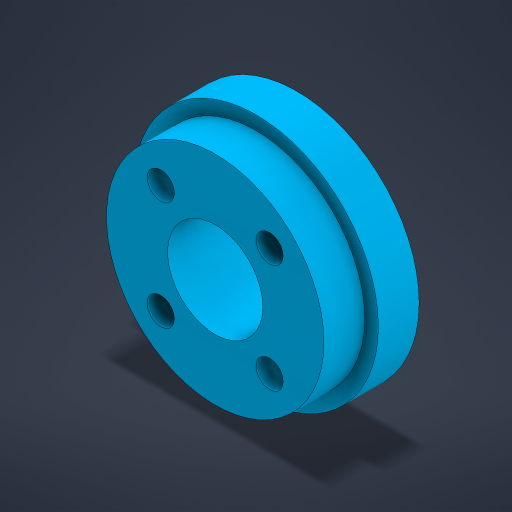
# Autodesk Inventor part: SecondStageArmClamp
Saved by Autodesk Inventor 2024 (Build 280153000, 153)
## iProperties
Created: 2024-01-28
Part Number: SecondStageArmClamp
Material: Generic
Document SubType Name: Modeling
Designer: avsar
Density: 1 g/cm^3
Appearance: Sky Blue Medium
Author: avsar
Autodesk Inventor part; units mm, degrees
ref_plane "YZ Plane" through (0, 0, 0) normal (1, 0, 0) x (0, 1, 0)
ref_plane "XZ Plane" through (0, 0, 0) normal (0, 1, 0) x (-1, 0, 0)
ref_plane "XY Plane" through (0, 0, 0) normal (0, 0, 1) x (1, 0, 0)
sketch "Sketch1" plane through (0, 0, 0) normal (0, 0, 1) x (1, 0, 0)
  circle A0 centre (0, 0) radius 18
  dimension "d0" = 36
  constraints: 1 centre point, 1 coincident
  measures "d0" diameter of A0
extrude "Extrusion1" add sketch "Sketch1" along normal blind 6
sketch "Sketch2" plane through (0, 0, 6) normal (0, 0, 1) x (1, 0, 0)
  circle A0 centre (0, 0) radius 16
  dimension "d3" = 32
  constraints: 1 centre point, 1 coincident
  measures "d3" diameter of A0
extrude "Extrusion2" add sketch "Sketch2" along normal blind 6
sketch "Sketch3" plane through (0, 0, 12) normal (0, 0, 1) x (1, 0, 0)
  circle A0 centre (0, 0) radius 7
  circle A1 centre (-8, 8) radius 2
  circle A2 centre (-8, -8) radius 2
  circle A3 centre (8, -8) radius 2
  circle A4 centre (8, 8) radius 2
  dimension "d6" = 14
  dimension "d7" = 4
  dimension "d8" = 8
  dimension "d9" = 8
  dimension "d12" = 360
  constraints: 5 centre point, 1 coincident, 9 other
  measures "d6" diameter of A0
  measures "d7" diameter of A1
  measures "d8" horizontal distance of A1.centre point (0, 0)
  measures "d9" horizontal distance of point (0, 0) A1.centre
extrude "Extrusion3" cut sketch "Sketch3" against normal through all
body "Solid1"
